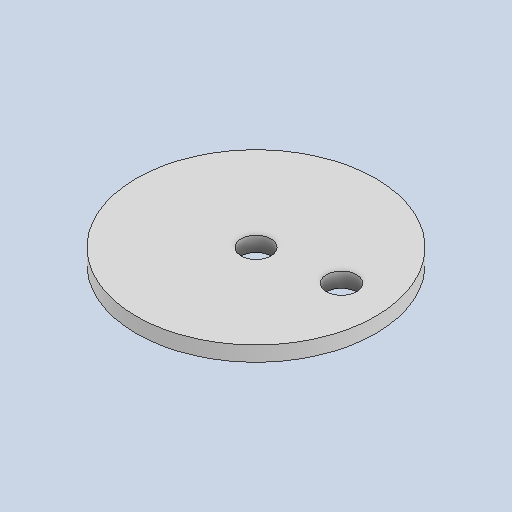
# Autodesk Inventor part: Prostavka
Saved by Autodesk Inventor 2023 (Build 270158000, 158)
## iProperties
Created: 2023-12-24
Part Number: Prostavka
Material: Типовые
Document SubType Name: Modeling
Designer: Dell
Density: 1 g/cm^3
Appearance: По умолчанию
Mass: 14.1356 g
Surface Area: 82.8674 cm^2
Volume: 14.1356 cm^3
Author: Dell
Autodesk Inventor part; units mm, degrees
ref_plane "YZ Plane" through (0, 0, 0) normal (1, 0, 0) x (0, 1, 0)
ref_plane "XZ Plane" through (0, 0, 0) normal (0, 1, 0) x (-1, 0, 0)
ref_plane "XY Plane" through (0, 0, 0) normal (0, 0, 1) x (1, 0, 0)
sketch "Эскиз1" plane through (0, 0, 0) normal (0, 1, 0) x (-1, 0, 0)
  circle A0 centre (0, 0) radius 32
  circle A1 centre (0, 0) radius 4
  dimension "d0" = 64
  dimension "d3" = 8
  constraints: 2 centre point, 2 coincident
  measures "d0" diameter of A0
  measures "d3" diameter of A1
extrude "Выдавливание2" add sketch "Эскиз1" along normal blind 4
sketch "Эскиз5" plane through (0, 4, 0) normal (0, 1, 0) x (1, 0, 0)
  arc A0 (-18.8207, 0.7432) -> (-20.681, -7.0375) centre (-19.7508, -3.1471) ccw projected
  arc A1 (-20.681, -7.0375) -> (-18.8207, 0.7432) centre (-19.7508, -3.1471) ccw projected
  arc A2 (20.681, 7.0375) -> (18.8207, -0.7432) centre (19.7508, 3.1471) ccw projected
  arc A3 (18.8207, -0.7432) -> (20.681, 7.0375) centre (19.7508, 3.1471) ccw projected
  arc A4 (4.0773, -15.8605) -> (2.217, -23.6412) centre (3.1471, -19.7508) ccw projected
  arc A5 (2.217, -23.6412) -> (4.0773, -15.8605) centre (3.1471, -19.7508) ccw projected
  arc A6 (-2.217, 23.6412) -> (-4.0773, 15.8605) centre (-3.1471, 19.7508) ccw projected
  arc A7 (-4.0773, 15.8605) -> (-2.217, 23.6412) centre (-3.1471, 19.7508) ccw projected
  point P0 (0, 0)
extrude "Выдавливание5" cut sketch "Эскиз5" against normal blind 10 contours A3 A2
